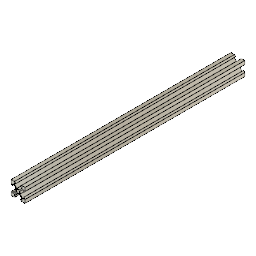
2020-315 only v2 (Autodesk Fusion 360 design; units mm, degrees)
Autodesk Fusion 360 part; units mm, degrees
sketch "Sketch1" plane through (0, 0, 0) normal (0, 1, 0) x (1, 0, 0)
  circle A0 centre (0, 0) radius 2.1
  line L0 (-6.56, 5.4993) -> (-8.2, 5.4993)
  line L1 (-8.2, 5.4993) -> (-8.2, 3.1)
  line L2 (-8.2, 3.1) -> (-10, 4.9)
  line L3 (-10, 4.9) -> (-10, 10)
  line L4 (-10, 10) -> (-4.9, 10)
  line L5 (-4.9, 10) -> (-3.1, 8.2)
  line L6 (-3.1, 8.2) -> (-5.4993, 8.2)
  line L7 (-5.4993, 8.2) -> (-5.4993, 6.56)
  line L8 (-5.4993, 6.56) -> (-1.7793, 2.84)
  line L9 (-6.56, 5.4993) -> (-2.84, 1.7793)
  line L10 (0, 0) -> (-10, 10) construction
  line L11 (0, 0) -> (0, 5) construction
  line L12 (0, 0) -> (-5, 0) construction
  line L13 (-2.84, 1.7793) -> (-2.84, 0)
  line L14 (-1.7793, 2.84) -> (0, 2.84)
  line L15 (-8.2, -3.1) -> (-10, -4.9)
  line L16 (-6.56, -5.4993) -> (-8.2, -5.4993)
  line L17 (-10, -4.9) -> (-10, -10)
  line L18 (-4.9, -10) -> (-3.1, -8.2)
  line L19 (-5.4993, -6.56) -> (-1.7793, -2.84)
  line L20 (-6.56, -5.4993) -> (-2.84, -1.7793)
  line L21 (-1.7793, -2.84) -> (0, -2.84)
  line L22 (-3.1, -8.2) -> (-5.4993, -8.2)
  line L23 (-8.2, -5.4993) -> (-8.2, -3.1)
  line L24 (-10, -10) -> (-4.9, -10)
  line L25 (-5.4993, -8.2) -> (-5.4993, -6.56)
  line L26 (-2.84, -1.7793) -> (-2.84, 0)
  line L27 (4.9, 10) -> (3.1, 8.2)
  line L28 (6.56, -5.4993) -> (8.2, -5.4993)
  line L29 (2.84, -1.7793) -> (2.84, 0)
  line L30 (6.56, -5.4993) -> (2.84, -1.7793)
  line L31 (10, 4.9) -> (10, 10)
  line L32 (1.7793, 2.84) -> (0, 2.84)
  line L33 (5.4993, -8.2) -> (5.4993, -6.56)
  line L34 (5.4993, -6.56) -> (1.7793, -2.84)
  line L35 (10, 10) -> (4.9, 10)
  line L36 (10, -4.9) -> (10, -10)
  line L37 (2.84, 1.7793) -> (2.84, 0)
  line L38 (3.1, 8.2) -> (5.4993, 8.2)
  line L39 (8.2, 3.1) -> (10, 4.9)
  line L40 (10, -10) -> (4.9, -10)
  line L41 (8.2, -3.1) -> (10, -4.9)
  line L42 (1.7793, -2.84) -> (0, -2.84)
  line L43 (5.4993, 6.56) -> (1.7793, 2.84)
  line L44 (6.56, 5.4993) -> (8.2, 5.4993)
  line L45 (4.9, -10) -> (3.1, -8.2)
  line L46 (6.56, 5.4993) -> (2.84, 1.7793)
  line L47 (8.2, 5.4993) -> (8.2, 3.1)
  line L48 (5.4993, 8.2) -> (5.4993, 6.56)
  line L49 (3.1, -8.2) -> (5.4993, -8.2)
  line L50 (8.2, -5.4993) -> (8.2, -3.1)
  line L51 (10, -4.9) -> (10, 4.9) construction
  point P0 (5, 0)
  dimension "d1" = 4.2
  dimension "d7" = 10
  dimension "d8" = 10
  dimension "d9" = 3.1
  dimension "d10" = 1.8
  dimension "d11" = 1.8
  dimension "d12" = 1.5
  dimension "d13" = 1.64
  dimension "d14" = 135
  dimension "d16" = 3.1
  dimension "d19" = 2.84
  dimension "d20" = 2.84
  dimension "d21" = 1.64
  constraint coincident A0.centre L10.start
  constraint perpendicular L0 L1
  constraint perpendicular L3 L4
  constraint parallel L2 L5
  constraint perpendicular L3 L6
  constraint perpendicular L6 L7
  constraint vertical L3
  constraint equal L8 L9
  constraint parallel L8 L10
  constraint vertical L11
  constraint perpendicular L11 L12
  constraint coincident L12 L13.end
  constraint perpendicular L12 L13
  constraint coincident L11 L14.end
  constraint perpendicular L11 L14
  constraint symmetric L8.end L9.end L10
  constraint symmetric L0.start L12 L16.start
  constraint symmetric L0.end L12 L16.end
  constraint symmetric L1.end L12 L15.start
  constraint symmetric L2.end L12 L15.end
  constraint symmetric L3.end L12 L17.end
  constraint symmetric L4.end L12 L18.start
  constraint symmetric L5.end L12 L18.end
  constraint symmetric L6.end L12 L22.end
  constraint symmetric L7.end L12 L19.start
  constraint symmetric L8.end L12 L19.end
  constraint symmetric L9.end L12 L20.end
  constraint symmetric L12 L13.end L26.end
  constraint symmetric L12 L14.end L21.end
  constraint symmetric L0.start L11 L44.start
  constraint symmetric L0.end L11 L44.end
  constraint symmetric L1.end L11 L39.start
  constraint symmetric L2.end L11 L31.start
  constraint symmetric L3.end L11 L31.end
  constraint symmetric L4.end L11 L27.start
  constraint symmetric L5.end L11 L27.end
  constraint symmetric L6.end L11 L38.end
  constraint symmetric L7.end L11 L43.start
  constraint symmetric L8.end L11 L32.start
  constraint symmetric L9.end L11 L37.start
  constraint symmetric L11 L12.end P0
  constraint symmetric L11 L13.end L29.end
  constraint symmetric L11 L14.end L32.end
  constraint symmetric L11 L16.end L28.end
  constraint symmetric L11 L15.start L41.start
  constraint symmetric L11 L17.end L36.end
  constraint symmetric L11 L22.end L33.start
  constraint symmetric L11 L20.end L29.start
  constraint symmetric L11 L15.end L36.start
  constraint symmetric L11 L19.end L34.end
  constraint symmetric L11 L19.start L33.end
  constraint symmetric L11 L18.end L45.end
  constraint symmetric L11 L18.start L40.end
  constraint symmetric L11 L16.start L28.start
  constraint symmetric L11 L21.end L42.end
  measures "d1" diameter of A0
  measures "d7" distance of A0.centre L4
  measures "d8" distance of A0.centre L3
  measures "d9" vertical distance of A0.centre L1.end
  measures "d10" distance of L1 L3
  measures "d11" distance of L4 L6
  measures "d12" distance of L8 L9
  measures "d13" distance of L6.end L7.end
  measures "d14" angle of L2 L3
  measures "d16" horizontal distance of A0.centre L5.end
  measures "d19" distance of L9.end L11
  measures "d20" vertical distance of A0.centre L8.end
  measures "d21" distance of L0.start L0.end
extrude "Extrude1" add sketch "Sketch1" along normal mid plane 315
equation "d9 = ( 6.2 / 2 ) * 1 mm"
equation "d11 = d10"
equation "d16 = d9"
equation "d19 = ( 5.68 / 2 ) * 1 mm"
equation "d20 = d19"
equation "d21 = d13"
